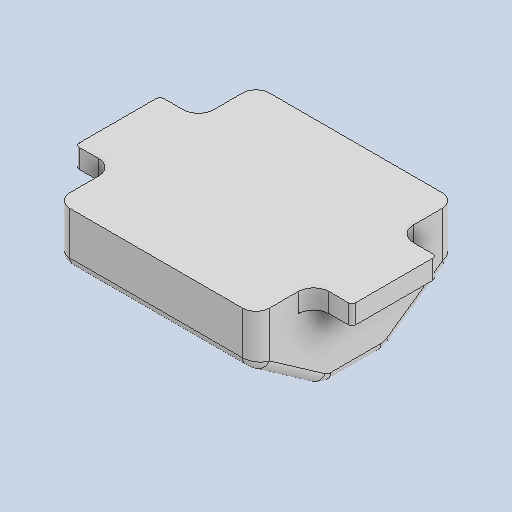
# Autodesk Inventor part: pinatel
Saved by Autodesk Inventor 2022 (Build 260153000, 153)
## iProperties
Created: 2025-01-07
Part Number: pinatel
Material: Типовые
Document SubType Name: Modeling
Designer: akap
Density: 1 g/cm^3
Appearance: По умолчанию
Author: akap
Autodesk Inventor part; units mm, degrees
ref_plane "YZ Plane" through (0, 0, 0) normal (1, 0, 0) x (0, 1, 0)
ref_plane "XZ Plane" through (0, 0, 0) normal (0, 1, 0) x (-1, 0, 0)
ref_plane "XY Plane" through (0, 0, 0) normal (0, 0, 1) x (1, 0, 0)
sketch "Эскиз1" plane through (0, 0, 0) normal (0, 1, 0) x (-1, 0, 0)
  line L0 (9.3708, 3) -> (9.3708, -3) projected
  line L1 (9.3708, -3) -> (9.3708, -4.5) projected
  arc A0 (8.3708, -5.5) -> (9.3708, -4.5) centre (8.3708, -4.5) ccw projected
  line L2 (8.3708, -5.5) -> (-0.6292, -5.5) projected
  arc A1 (-1.6292, -4.5) -> (-0.6292, -5.5) centre (-0.6292, -4.5) ccw projected
  line L3 (-1.6292, -4.5) -> (-1.6292, -3) projected
  arc A2 (-1.6292, -3) -> (-2.1292, -2.5) centre (-2.1292, -3) ccw projected
  line L4 (-3.1292, -2.5) -> (-2.1292, -2.5) projected
  arc A3 (-3.6292, -2) -> (-3.1292, -2.5) centre (-3.1292, -2) ccw projected
  line L5 (-3.6292, 2) -> (-3.6292, -2) projected
  arc A4 (-3.1292, 2.5) -> (-3.6292, 2) centre (-3.1292, 2) ccw projected
  line L6 (-2.1292, 2.5) -> (-3.1292, 2.5) projected
  arc A5 (-2.1292, 2.5) -> (-1.6292, 3) centre (-2.1292, 3) ccw projected
  line L7 (-1.6292, 3) -> (-1.6292, 4.5) projected
  arc A6 (-0.6292, 5.5) -> (-1.6292, 4.5) centre (-0.6292, 4.5) ccw projected
  line L8 (-0.6292, 5.5) -> (8.3708, 5.5) projected
  arc A7 (9.3708, 4.5) -> (8.3708, 5.5) centre (8.3708, 4.5) ccw projected
  line L9 (9.3708, 4.5) -> (9.3708, 3) projected
  arc A8 (6.8708, 1.5) -> (5.3708, 3) centre (5.3708, 1.5) ccw projected
  line L10 (2.3708, 3) -> (5.3708, 3) projected
  arc A9 (2.3708, 3) -> (0.8708, 1.5) centre (2.3708, 1.5) ccw projected
  line L11 (0.8708, -1.5) -> (0.8708, 1.5) projected
  arc A10 (0.8708, -1.5) -> (2.3708, -3) centre (2.3708, -1.5) ccw projected
  line L12 (5.3708, -3) -> (2.3708, -3) projected
  arc A11 (5.3708, -3) -> (6.8708, -1.5) centre (5.3708, -1.5) ccw projected
  line L13 (6.8708, 1.5) -> (6.8708, -1.5) projected
  arc A12 (9.8708, -2.5) -> (9.3708, -3) centre (9.8708, -3) ccw projected
  line L14 (9.3708, 3) -> (9.3708, -3) projected
  arc A13 (9.3708, 3) -> (9.8708, 2.5) centre (9.8708, 3) ccw projected
  line L15 (10.8708, 2.5) -> (9.8708, 2.5) projected
  arc A14 (11.3708, 2) -> (10.8708, 2.5) centre (10.8708, 2) ccw projected
  line L16 (11.3708, -2) -> (11.3708, 2) projected
  arc A15 (10.8708, -2.5) -> (11.3708, -2) centre (10.8708, -2) ccw projected
  line L17 (9.8708, -2.5) -> (10.8708, -2.5) projected
  line L18 (9.0708, 3) -> (9.0708, 4.5)
  arc A16 (9.0708, 4.5) -> (8.3708, 5.2) centre (8.3708, 4.5) ccw
  line L19 (8.3708, 5.2) -> (-0.6292, 5.2)
  arc A17 (-0.6292, 5.2) -> (-1.3292, 4.5) centre (-0.6292, 4.5) ccw
  line L20 (-1.3292, 4.5) -> (-1.3292, 3)
  arc A18 (-2.1292, 2.2) -> (-1.3292, 3) centre (-2.1292, 3) ccw
  line L21 (-2.1292, 2.2) -> (-3.1292, 2.2)
  arc A19 (-3.1292, 2.2) -> (-3.3292, 2) centre (-3.1292, 2) ccw
  line L22 (-3.3292, 2) -> (-3.3292, -2)
  arc A20 (-3.3292, -2) -> (-3.1292, -2.2) centre (-3.1292, -2) ccw
  line L23 (-3.1292, -2.2) -> (-2.1292, -2.2)
  arc A21 (-1.3292, -3) -> (-2.1292, -2.2) centre (-2.1292, -3) ccw
  line L24 (-1.3292, -3) -> (-1.3292, -4.5)
  arc A22 (-1.3292, -4.5) -> (-0.6292, -5.2) centre (-0.6292, -4.5) ccw
  line L25 (-0.6292, -5.2) -> (8.3708, -5.2)
  arc A23 (8.3708, -5.2) -> (9.0708, -4.5) centre (8.3708, -4.5) ccw
  line L26 (9.0708, -4.5) -> (9.0708, -3)
  arc A24 (9.0708, 3) -> (9.8708, 2.2) centre (9.8708, 3) ccw
  line L27 (9.8708, 2.2) -> (10.8708, 2.2)
  arc A25 (11.0708, 2) -> (10.8708, 2.2) centre (10.8708, 2) ccw
  line L28 (11.0708, 2) -> (11.0708, -2)
  arc A26 (10.8708, -2.2) -> (11.0708, -2) centre (10.8708, -2) ccw
  line L29 (10.8708, -2.2) -> (9.8708, -2.2)
  arc A27 (9.8708, -2.2) -> (9.0708, -3) centre (9.8708, -3) ccw
  point P0 (0, 0)
  dimension "d0" = 0.3
  dimension "d1" = 0.3
  constraints: 24 end point, 24 point on circle, 12 centre point, 22 other
  measures "d0" distance between parallel lines of L2 L25
  measures "d1" distance between parallel lines of L17 L29
extrude "Выдавливание1" add sketch "Эскиз1" along normal blind 1 contours A24 L27 A25 L28 A26 L29 A27 L0 | L0 A27 L26 A23 L25 A22 L24 A21 L23 A20 L22 A19 L21 A18 L20 A17 L19 A16 L18 A24 | L13 A11 L12 A10 L11 A9 L10 A8
sketch "Эскиз2" plane through (0, 0, 0) normal (0, -1, 0) x (1, 0, 0)
  arc A0 (-8.3708, 5.2) -> (-9.0708, 4.5) centre (-8.3708, 4.5) ccw projected
  line L0 (-9.0708, 3) -> (-9.0708, 4.5) projected
  arc A1 (-9.8708, 2.2) -> (-9.0708, 3) centre (-9.8708, 3) ccw projected
  line L1 (-10.8708, 2.2) -> (-9.8708, 2.2) projected
  arc A2 (-10.8708, 2.2) -> (-11.0708, 2) centre (-10.8708, 2) ccw projected
  line L2 (-11.0708, -2) -> (-11.0708, 2) projected
  arc A3 (-11.0708, -2) -> (-10.8708, -2.2) centre (-10.8708, -2) ccw projected
  line L3 (-9.8708, -2.2) -> (-10.8708, -2.2) projected
  arc A4 (-9.0708, -3) -> (-9.8708, -2.2) centre (-9.8708, -3) ccw projected
  line L4 (-9.0708, -4.5) -> (-9.0708, -3) projected
  arc A5 (-9.0708, -4.5) -> (-8.3708, -5.2) centre (-8.3708, -4.5) ccw projected
  line L5 (0.6292, -5.2) -> (-8.3708, -5.2) projected
  arc A6 (0.6292, -5.2) -> (1.3292, -4.5) centre (0.6292, -4.5) ccw projected
  line L6 (1.3292, -3) -> (1.3292, -4.5) projected
  arc A7 (2.1292, -2.2) -> (1.3292, -3) centre (2.1292, -3) ccw projected
  line L7 (3.1292, -2.2) -> (2.1292, -2.2) projected
  arc A8 (3.1292, -2.2) -> (3.3292, -2) centre (3.1292, -2) ccw projected
  line L8 (3.3292, 2) -> (3.3292, -2) projected
  arc A9 (3.3292, 2) -> (3.1292, 2.2) centre (3.1292, 2) ccw projected
  line L9 (2.1292, 2.2) -> (3.1292, 2.2) projected
  arc A10 (1.3292, 3) -> (2.1292, 2.2) centre (2.1292, 3) ccw projected
  line L10 (1.3292, 4.5) -> (1.3292, 3) projected
  arc A11 (1.3292, 4.5) -> (0.6292, 5.2) centre (0.6292, 4.5) ccw projected
  line L11 (-8.3708, 5.2) -> (0.6292, 5.2) projected
  arc A12 (-9.8708, 2.2) -> (-9.0708, 3) centre (-9.8708, 3) ccw projected
  line L12 (-9.0708, -3) -> (-9.0708, 3)
  line L13 (1.3292, 3) -> (1.3292, -3)
  point P0 (0, 0)
  constraints: 4 end point, 2 tangent, 1 vertical
extrude "Выдавливание2" add sketch "Эскиз2" along normal blind 4 contours L11 A11 L10 L13 L6 A6 L5 A5 L4 L12 L0 A0
sketch "Эскиз3" plane through (-9.0708, 0, -3) normal (-1, 0, 0) x (0, 0, 1)
  line L0 (0, 0) -> (0, 1) projected
  line L1 (-1.5, 1) -> (0, 1) projected
  line L2 (-1.5, -4) -> (-1.5, 1) projected
  line L3 (7.5, -4) -> (-1.5, -4) projected
  line L4 (7.5, 1) -> (7.5, -4) projected
  line L5 (6, 1) -> (7.5, 1) projected
  line L6 (6, 0) -> (6, 1) projected
  line L7 (0, 0) -> (6, 0) projected
  line L8 (7.5, 1) -> (8.2, 1) projected
  line L9 (7.5, 1) -> (7.5, -4) projected
  line L10 (-1.5, -4) -> (-1.5, 1) projected
  line L11 (-2.2, 1) -> (-1.5, 1) projected
  line L12 (-2.2, -4) -> (-2.2, 1) projected
  line L13 (-1.5, -4) -> (-2.2, -4) projected
  line L14 (8.2, 1) -> (7.5, 1) projected
  line L15 (8.2, -1.5) -> (4.6296, -4)
  line L16 (7.5, -4) -> (-1.5, -4) projected
  line L17 (-1.5, 1) -> (-2.2, 1) projected
  line L18 (-2.2, 1) -> (-2.2, -1.5)
  line L19 (-2.2, -4) -> (-2.2, 1) projected
  line L20 (-2.2, -1.5) -> (1.3704, -4)
  line L21 (7.5, 1) -> (7.5, -4) projected
  line L22 (8.2, -4) -> (8.2, 1) projected
  line L23 (7.5, -4) -> (8.2, -4) projected
  line L24 (8.2, 1) -> (8.2, -1.5)
  point P0 (3, 0)
  point P1 (-2.2, -1.5)
  dimension "d8" = 2.5
  dimension "d9" = 35
  dimension "d10" = 35
  dimension "d14" = 2.5
  constraints: 8 end point, 3 midpoint, 2 point on line
  measures "d8" distance of L11.start L18.end
  measures "d9" angle of L3 L20
  measures "d10" angle of L3 L15
  measures "d14" distance of L22.end L24.end
extrude "Выдавливание3" cut sketch "Эскиз3" against normal blind 15 contours L20 L3 L2 | L2 L13 L12 L20 | L15 L22 L23 L4 | L4 L3 L15
fillet "Сопряжение2" radius 1 2 edges at (-3.8708, -4, -1.6296) (-3.8708, -4, 1.6296)
fillet "Сопряжение3" radius 0.5 8 edges at (-9.0708, -2.9046, 3.194) (-8.8657, -1.6436, 4.995) (-3.8708, -1.5, 5.2) (1.1242, -1.6436, 4.995) (1.3292, -2.9046, 3.194) (1.1242, -1.6436, -4.995) (-3.8708, -1.5, -5.2) (-8.8657, -1.6436, -4.995)
